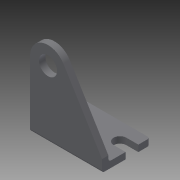
# Autodesk Inventor part: D-14826
Saved by Autodesk Inventor 2014 (Build 180170000, 170)
## iProperties
Created: 2014-01-18
Part Number: D-14826
Material: Steel
Catalog Web Link: www.cadenas.de
Description: Pivot Bracket for Original Line Cylinders - Right-
Vendor: BIMBA
Document SubType Name: Standard Catalog Part
Designer: Andrew Toennies
Manufacturer: BIMBA
Density: 1 g/cm^3
Appearance: Steel
Category: PARTsolutions
Company: BIMBA
PSOL_IDENT_0: {$CADENAS_DATA\23d-libs\bimba\bimba\bimba_imperial\bimba_full_line\original_line_cylinders\accessori
PSOL_IDENT_1: es\pivot_bracket_right.prj},199 {VTYP=3D},{NB=D-14826},{LINA=D-14826},{NN=Pivot Bracket for Original
PSOL_IDENT_2: Line Cylinders - Right},{DATE=06.12.2011 08:05:39},{GEOMDATE=06.12.2011 08:05:00},{VERSION=},{LINEI
PSOL_IDENT_3: D=40},{LINESUBID=-1},{WBVAR=}  {NB=D-14826},{LINA=D-14826},{KT=DUMMY},{PN=D-14826},{MAT=Zinc-Plated
PSOL_IDENT_4: Carbon Steel},{CD=0},{L=1.50000000},{L1=1.00000000},{L2=0.50000000},{L3=0.75000000},{L5=0.37500000},
PSOL_IDENT_5: {L6=0.13450000},{H=1.75000000},{H1=0.25000000},{H2=1.37500000},{H22=1.375},{W=1.00000000},{W1=0.2660
PSOL_IDENT_6: 0000},{W2=0.62500000},{R1=0.13300000},{R2=0.37500000},{R3=0.05000000},{D1=0.37750000},{C=1}
CNS_NN: Pivot Bracket for Original Line Cylinders - Right
CNS_NB: D-14826
CNS_NBSYN: $PN.
CNS_LINA: D-14826
CNS_PN: D-14826
CNS_MAT: Zinc-Plated Carbon Steel
CNS_CD: 0
CNS_L: 1.50000000
CNS_L1: 1.00000000
CNS_L2: 0.50000000
CNS_L3: 0.75000000
CNS_L5: 0.37500000
CNS_L6: 0.13450000
CNS_H: 1.75000000
CNS_H1: 0.25000000
CNS_H2: 1.37500000
CNS_H22: 1.375
CNS_W: 1.00000000
CNS_W1: 0.26600000
CNS_W2: 0.62500000
CNS_R1: 0.13300000
CNS_R2: 0.37500000
CNS_R3: 0.05000000
CNS_D1: 0.37750000
CNS_C: 1
SUPPLIER: BIMBA
ARTICLENO: D-14826
BOMINFO: D-14826
CREATOR: CADENAS GmbH
Title: D-14826
Author: Cadenas PARTsolutions
Autodesk Inventor part; units mm, degrees
ref_plane "YZ Plane" through (0, 0, 0) normal (1, 0, 0) x (0, 1, 0)
ref_plane "XZ Plane" through (0, 0, 0) normal (0, 1, 0) x (-1, 0, 0)
ref_plane "XY Plane" through (0, 0, 0) normal (0, 0, 1) x (1, 0, 0)
sketch "Sketch_1" plane through (0, 0, 0) normal (1, 0, 0) x (0, 1, 0)
  line L0 (44.45, 0) -> (1.27, 0)
  arc A0 (1.27, 0) -> (0, -1.27) centre (1.27, -1.27) ccw
  line L1 (0, -1.27) -> (0, -25.4)
  line L2 (0, -25.4) -> (3.4163, -25.4)
  line L3 (3.4163, -25.4) -> (3.4163, -4.6863)
  arc A1 (4.6863, -3.4163) -> (3.4163, -4.6863) centre (4.6863, -4.6863) ccw
  line L4 (4.6863, -3.4163) -> (44.45, -3.4163)
  line L5 (44.45, -3.4163) -> (44.45, 0)
  constraints: 12 end point, 4 point on circle, 2 centre point
extrude "Extrusion1" add sketch "Sketch_1" along normal blind 38.1
sketch "Sketch_2" plane through (0, 0, 0) normal (0, 0, 1) x (1, 0, 0)
  line L0 (-38.1, -44.45) -> (57.15, -44.45)
  line L1 (57.15, -44.45) -> (57.15, 66.675)
  line L2 (57.15, 66.675) -> (-38.1, 66.675)
  line L3 (-38.1, 66.675) -> (-38.1, -44.45)
  line L4 (0, 0) -> (38.1, 0)
  line L5 (38.1, 0) -> (38.1, 6.35)
  line L6 (38.1, 6.35) -> (17.6579, 39.8829)
  arc A0 (17.6579, 39.8829) -> (0, 34.925) centre (9.525, 34.925) ccw
  line L7 (0, 34.925) -> (0, 0)
  constraints: 16 end point, 2 point on circle, 1 centre point
extrude "Extrusion2" cut sketch "Sketch_2" against normal blind 25.4
sketch "Sketch3" plane through (0, 1.27, 0) normal (0, 0, 1) x (1, 0, 0)
  point P0 (9.525, 33.655)
hole "Hole1" at (9.525, 34.925, 0) direction (0, 0, -1) diameter 9.5885 depth 3.4163
sketch "Sketch4" plane through (0, 0, -25.4) normal (0, -1, 0) x (1, 0, 0)
  point P0 (6.35, 9.525)
hole "Hole2" at (6.35, 0, -15.875) direction (0, 1, 0) diameter 6.7564 depth 3.4163
sketch "Sketch5" plane through (0, 0, -25.4) normal (0, -1, 0) x (1, 0, 0)
  point P0 (31.75, 9.525)
hole "Hole3" at (31.75, 0, -15.875) direction (0, 1, 0) diameter 6.7564 depth 3.4163
sketch "Sketch_6" plane through (0, 0, 0) normal (0, 1, 0) x (-1, 0, 0)
  line L0 (0, -19.2532) -> (0, -12.4968)
  line L1 (0, -12.4968) -> (-6.35, -12.4968)
  line L2 (-6.35, -12.4968) -> (-6.35, -19.2532)
  line L3 (-6.35, -19.2532) -> (0, -19.2532)
  constraints: 8 end point
sketch "Sketch_7" plane through (0, 0, 0) normal (0, 1, 0) x (-1, 0, 0)
  line L0 (-31.75, -19.2532) -> (-31.75, -12.4968)
  line L1 (-31.75, -12.4968) -> (-38.1, -12.4968)
  line L2 (-38.1, -12.4968) -> (-38.1, -19.2532)
  line L3 (-38.1, -19.2532) -> (-31.75, -19.2532)
  constraints: 8 end point
extrude "Extrusion3" cut sketch "Sketch_6" along normal blind 3.4163
extrude "Extrusion4" cut sketch "Sketch_7" along normal blind 3.4163
sketch "Sketch_8" plane through (0, 0, 0) normal (0, 1, 0) x (-1, 0, 0)
  line L0 (0, -38.1) -> (0, -24.13)
  arc A0 (-1.27, -25.4) -> (0, -24.13) centre (-1.27, -24.13) ccw
  line L1 (-1.27, -25.4) -> (-36.83, -25.4)
  arc A1 (-38.1, -24.13) -> (-36.83, -25.4) centre (-36.83, -24.13) ccw
  line L2 (-38.1, -24.13) -> (-38.1, -38.1)
  line L3 (-38.1, -38.1) -> (0, -38.1)
  constraints: 8 end point, 4 point on circle, 2 centre point
extrude "Extrusion5" cut sketch "Sketch_8" along normal blind 3.4163
ref_plane "to_dummy_R_XY" through (0, 0, 0) normal (0, 0, 1) x (1, 0, 0)
ref_plane "to_dummy_R_YZ" through (0, 0, 0) normal (1, 0, 0) x (0, 1, 0)
ref_plane "to_dummy_R_ZX" through (0, 0, 0) normal (0, 1, 0) x (0, 0, 1)
ref_plane "to_pin_R_XY" through (9.525, 34.925, 0) normal (0, 0, 1) x (1, 0, 0)
ref_plane "to_pin_R_YZ" through (9.525, 34.925, 0) normal (1, 0, 0) x (0, 1, 0)
ref_plane "to_pin_R_ZX" through (9.525, 34.925, 0) normal (0, 1, 0) x (0, 0, 1)
body "Solid1"
